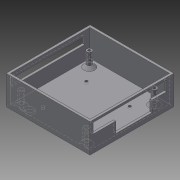
# Autodesk Inventor part: nuccase
Saved by Autodesk Inventor 2015 (Build 190159000, 159)
## iProperties
Created: 2016-10-24
Part Number: nuccase
Material: Generic
Document SubType Name: Modeling
Designer: Bardo91
Density: 1 g/cm^3
Appearance: Default
Author: Bardo91
Autodesk Inventor part; units mm, degrees
ref_plane "YZ Plane" through (0, 0, 0) normal (1, 0, 0) x (0, 1, 0)
ref_plane "XZ Plane" through (0, 0, 0) normal (0, 1, 0) x (-1, 0, 0)
ref_plane "XY Plane" through (0, 0, 0) normal (0, 0, 1) x (1, 0, 0)
sketch "Sketch1" plane through (0, 0, 0) normal (0, 0, 1) x (1, 0, 0)
  line L0 (0, 0) -> (0, 110)
  line L1 (0, 110) -> (110, 110)
  line L2 (110, 110) -> (110, 0)
  line L3 (110, 0) -> (0, 0)
  dimension "d0" = 110
  dimension "d1" = 110
  constraints: 8 end point, 3 perpendicular, 1 vertical
  measures "d0" distance of L0.start L0.end
  measures "d1" distance of L0.end L1.end
extrude "Extrusion1" add sketch "Sketch1" along normal blind 3
sketch "Sketch2" plane through (0, 0, 0) normal (0, 0, -1) x (-1, 0, 0)
  line L0 (0, 0) -> (3, 0)
  line L1 (3, 0) -> (3, 113)
  line L2 (3, 113) -> (-113, 113)
  line L3 (-113, 113) -> (-113, -3)
  line L4 (-113, -3) -> (3, -3)
  line L5 (3, -3) -> (3, 0)
  line L6 (-110, 110) -> (0, 110)
  line L7 (0, 110) -> (0, 0)
  line L8 (0, 0) -> (-110, 0)
  line L9 (-110, 0) -> (-110, 110)
  dimension "d4" = 3
  dimension "d5" = 113
  dimension "d6" = 116
  dimension "d7" = 116
  constraints: 20 end point, 5 perpendicular, 2 horizontal, 2 parallel, 1 point on line, 1 vertical
  measures "d4" distance of L0.start L0.end
  measures "d5" distance of L0.end L1.end
  measures "d6" distance of L1.end L2.end
  measures "d7" distance of L2.end L3.end
extrude "Extrusion2" add sketch "Sketch2" against normal blind 40
sketch "Sketch3" plane through (0, 0, 3) normal (0, 0, 1) x (1, 0, 0)
  line L0 (110, 0) -> (0, 0) projected
  line L1 (55, 0) -> (55, 5)
  line L2 (55, 5) -> (10, 5)
  line L3 (55, 5) -> (100, 5)
  line L4 (100, 5) -> (100, 99)
  line L5 (100, 99) -> (10, 99)
  line L6 (10, 99) -> (10, 5)
  circle A0 centre (10, 5) radius 3.5
  circle A1 centre (10, 99) radius 3.5
  circle A2 centre (100, 99) radius 3.5
  circle A3 centre (100, 5) radius 3.5
  dimension "d10" = 5
  dimension "d11" = 45
  dimension "d12" = 45
  dimension "d13" = 94
  dimension "d14" = 90
  dimension "d15" = 7
  dimension "d16" = 7
  dimension "d17" = 7
  dimension "d18" = 7
  constraints: 12 end point, 4 centre point, 4 coincident, 3 perpendicular, 1 horizontal, 1 midpoint, 1 vertical
  measures "d10" distance of L1.start L1.end
  measures "d11" distance of L1.end L2.end
  measures "d12" distance of L1.end L3.end
  measures "d13" distance of L3.end L4.end
  measures "d14" distance of L4.end L5.end
  measures "d15" diameter of A0
  measures "d16" diameter of A1
  measures "d17" diameter of A2
  measures "d18" diameter of A3
extrude "Extrusion3" add sketch "Sketch3" along normal blind 20 contours A0 L6 L2 | L2 L6 A0 | A3 L4 L3 | L3 L4 A3 | A1 L5 L6 | L6 L5 A1 | A2 L5 L4 | L4 L5 A2
sketch "Sketch4" plane through (10, 99, 23) normal (0, 0, 1) x (1, 0, 0)
  circle A0 centre (0, 0) radius 1.75
  circle A1 centre (90, 0) radius 3.5 projected
  circle A2 centre (90, 0) radius 1.75
  circle A3 centre (90, -94) radius 3.5 projected
  circle A4 centre (90, -94) radius 1.75
  circle A5 centre (0, -94) radius 3.5 projected
  circle A6 centre (0, -94) radius 1.75
  point P0 (-10, -99)
  point P1 (90, -99)
  point P2 (0, -99)
  dimension "d21" = 3.5
  dimension "d22" = 3.5
  dimension "d23" = 3.5
  constraints: 4 centre point, 3 coincident, 2 vertical alignment
  measures "d21" diameter of A0
  measures "d22" diameter of A2
  measures "d23" diameter of A4
extrude "Extrusion4" cut sketch "Sketch4" against normal through all contours A0 | A2 | A4 | A6
sketch "Sketch5" plane through (0, 0, 3) normal (0, 0, 1) x (1, 0, 0)
  line L0 (110, 0) -> (0, 0) projected
  line L1 (55, 0) -> (55, 20)
  line L2 (55, 20) -> (85, 20)
  line L3 (85, 20) -> (85, 80)
  line L4 (85, 80) -> (25, 80)
  line L5 (25, 80) -> (25, 20)
  circle A0 centre (25, 20) radius 1.75
  circle A1 centre (25, 80) radius 1.75
  circle A2 centre (85, 80) radius 1.75
  circle A3 centre (85, 20) radius 1.75
  dimension "d26" = 20
  dimension "d27" = 30
  dimension "d28" = 60
  dimension "d29" = 60
  dimension "d30" = 3.5
  dimension "d31" = 3.5
  dimension "d32" = 3.5
  dimension "d33" = 3.5
  constraints: 10 end point, 4 centre point, 4 coincident, 4 perpendicular, 1 midpoint, 1 point on line, 1 vertical
  measures "d26" distance of L1.start L1.end
  measures "d27" distance of L1.end L2.end
  measures "d28" distance of L2.end L3.end
  measures "d29" distance of L3.end L4.end
  measures "d30" diameter of A0
  measures "d31" diameter of A1
  measures "d32" diameter of A2
  measures "d33" diameter of A3
extrude "Extrusion5" cut sketch "Sketch5" against normal through all
chamfer "Chamfer1" distance 4 angle 45 4 edges at (6.5, 99, 3) (96.5, 99, 3) (6.5, 5, 3) (96.5, 5, 3)
sketch "Sketch6" plane through (113, -3, 0) normal (1, 0, 0) x (0, 0, -1)
  line L0 (-23, 105.5) -> (-23, 98.5) projected
  line L1 (-23, 105.738) -> (-37, 105.738)
  line L2 (-23, 105.738) -> (-9, 105.738) construction
  line L3 (-23, 11.5) -> (-23, 4.5) projected
  line L4 (-23, 4.3379) -> (-37, 4.3379)
  line L5 (-23, 4.3379) -> (-9, 4.3379) construction
  line L6 (-37, 4.3379) -> (-37, 105.738)
  line L7 (-23, 105.738) -> (-23, 85.738)
  line L8 (-23, 85.738) -> (-8, 85.738)
  line L9 (-8, 85.738) -> (-8, 35.738)
  line L10 (-8, 35.738) -> (-23, 35.738)
  line L11 (-23, 35.738) -> (-23, 4.3379)
  point P0 (0, 3)
  dimension "d39" = 14
  dimension "d40" = 180
  dimension "d41" = 14
  dimension "d42" = 180
  dimension "d43" = 20
  dimension "d44" = 15
  dimension "d45" = 50
  constraints: 20 end point, 5 perpendicular, 3 point on line, 2 collinear, 2 horizontal, 1 parallel
  measures "d39" distance of L1.start L1.end
  measures "d40" angle of L1 L2
  measures "d41" distance of L4.start L4.end
  measures "d42" angle of L4 L5
  measures "d43" distance of L1.start L7.end
  measures "d44" distance of L7.end L8.end
  measures "d45" distance of L8.end L9.end
extrude "Extrusion6" cut sketch "Sketch6" against normal up to surface (3 mm away)
sketch "Sketch7" plane through (-3, -3, 0) normal (-1, 0, 0) x (0, 0, 1)
  line L0 (23, 105.738) -> (33, 105.738)
  line L1 (33, 105.738) -> (33, 5.738)
  line L2 (33, 5.738) -> (23, 5.738)
  line L3 (23, 5.738) -> (23, 105.738)
  point P0 (0, 3)
  dimension "d48" = 10
  dimension "d49" = 100
  constraints: 8 end point, 2 parallel, 1 horizontal, 1 perpendicular
  measures "d48" distance of L1.end L2.end
  measures "d49" distance of L0.end L1.end
extrude "Extrusion7" cut sketch "Sketch7" against normal up to surface (3 mm away)
sketch "Sketch8" plane through (0, 0, 0) normal (0, 0, -1) x (-1, 0, 0)
  circle A0 centre (-10, 5) radius 1.75 projected
  line L0 (-10, 5) -> (-20, 5)
  line L1 (-20, 5) -> (-20, 7)
  line L2 (-20, 5) -> (-18, 5) construction
  circle A1 centre (-20, 7) radius 5
  point P0 (0, 0)
  dimension "d52" = 10
  dimension "d53" = 2
  dimension "d54" = 90
  dimension "d55" = 10
  constraints: 6 end point, 2 horizontal, 1 centre point, 1 coincident, 1 perpendicular, 1 vertical
  measures "d52" distance of L0.start L0.end
  measures "d53" distance of L0.end L1.end
  measures "d54" angle of L2 L1
  measures "d55" diameter of A1
extrude "Extrusion8" cut sketch "Sketch8" against normal blind 20 contours A1
equation "\"d15\" = d16"
equation "\"d17\" = d16"
equation "\"d18\" = d16"
body "Solid1"
